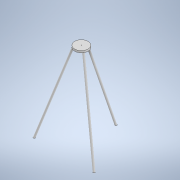
# Autodesk Inventor part: tripod
Saved by Autodesk Inventor 2021.1 (Build 251245010, 245A)
## iProperties
Created: 2020-11-06
Part Number: tripod
Material: Generic
Document SubType Name: Modeling
Designer: robst
Density: 1 g/cm^3
Appearance: Default
Author: robst
Autodesk Inventor part; units mm, degrees
ref_plane "YZ Plane" through (0, 0, 0) normal (1, 0, 0) x (0, 1, 0)
ref_plane "XY Plane" through (0, 0, 0) normal (0, 0, 1) x (1, 0, 0)
sketch "Sketch3" plane through (0, 0, 0) normal (0, 1, 0) x (-1, 0, 0)
  circle A0 centre (0, -457.2) radius 12.7
  point P0 (0, 0)
  dimension "d16" = 25.4
  dimension "d17" = 457.2
  constraints: 1 centre point
  measures "d16" diameter of A0
  measures "d17" distance of A0.centre point (0, 0)
ref_plane "Work Plane3" through (0, 1117.6, 0) normal (0, 1, 0) x (-1, 0, 0)
sketch "Sketch4" plane through (0, 1117.6, 0) normal (0, 1, 0) x (-1, 0, 0)
  circle A0 centre (0, -76.2) radius 12.7
  point P0 (0, 0)
  dimension "d19" = 76.2
  dimension "d20" = 25.4
  constraints: 1 centre point
  measures "d19" distance of A0.centre point (0, 0)
  measures "d20" diameter of A0
loft "Loft2" add profiles "Sketch3", "Sketch4"
pattern_circular "Circular Pattern1" count 3 over 360 about axis through (0, -10, 0) along (0, 1, 0) of "Loft2"
sketch "Sketch5" plane through (0, 1117.6, 0) normal (0, 1, 0) x (-1, 0, 0)
  circle A0 centre (0, 0) radius 88.9
  dimension "d28" = 177.8
  constraints: 1 centre point, 1 coincident
  measures "d28" diameter of A0
extrude "Extrusion1" add sketch "Sketch5" along normal blind 25.4
sketch "Sketch6" plane through (0, 1143, 0) normal (0, 1, 0) x (1, 0, 0)
  circle A0 centre (0, 0) radius 3.175
  dimension "d31" = 6.35
  constraints: 1 centre point, 1 coincident
  measures "d31" diameter of A0
extrude "Extrusion2" cut sketch "Sketch6" against normal through all
body "Solid2"
